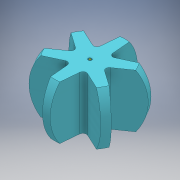
# Autodesk Inventor part: Dispensing Gear V2
Saved by Autodesk Inventor 2017 (Build 210142000, 142)
## iProperties
Created: 2018-12-12
Part Number: Dispensing Gear V2
Material: Generic
Document SubType Name: Modeling
Designer: Matt
Density: 1 g/cm^3
Appearance: Cadet Blue
Author: Matt
Autodesk Inventor part; units mm, degrees
ref_plane "YZ Plane" through (0, 0, 0) normal (1, 0, 0) x (0, 1, 0)
ref_plane "XZ Plane" through (0, 0, 0) normal (0, 1, 0) x (-1, 0, 0)
ref_plane "XY Plane" through (0, 0, 0) normal (0, 0, 1) x (1, 0, 0)
sketch "Sketch6" plane through (0, 0, 0) normal (0, 0, 1) x (1, 0, 0)
  circle A0 centre (0, 0) radius 2.75
  line L0 (0, 0) -> (0, 125)
  line L1 (0, 0) -> (108.2532, 62.5)
  line L2 (0, 0) -> (125, 0) construction
  line L3 (0, 0) -> (18.8687, 32.6815)
  line L4 (0, 0) -> (37.7374, 0) construction
  line L5 (108.2532, 62.5) -> (9.497, 16.4492)
  line L6 (108.2532, 62.5) -> (217.2186, 62.5) construction
  line L7 (9.497, 16.4492) -> (0, 125)
  line L8 (0, 125) -> (-9.497, 16.4492)
  line L9 (-9.497, 16.4492) -> (-108.2532, 62.5)
  line L10 (-108.2532, 62.5) -> (-18.9939, 0)
  line L11 (-18.9939, 0) -> (-108.2532, -62.5)
  line L12 (-108.2532, -62.5) -> (-9.497, -16.4492)
  line L13 (-9.497, -16.4492) -> (0, -125)
  line L14 (0, -125) -> (9.497, -16.4492)
  line L15 (9.497, -16.4492) -> (108.2532, -62.5)
  line L16 (108.2532, -62.5) -> (18.9939, 0)
  line L17 (18.9939, 0) -> (108.2532, 62.5)
  dimension "d21" = 5.5
  dimension "d22" = 125
  dimension "d23" = 30
  dimension "d24" = 60
  dimension "d25" = 155
  dimension "d28" = 360
  constraints: 36 end point, 3 equal length, 3 horizontal, 1 centre point, 1 coincident, 1 point on line, 1 vertical, 31 other
  measures "d21" diameter of A0
  measures "d22" distance of L0.start L0.end
  measures "d23" angle of L2 L1
  measures "d24" angle of L4 L3
  measures "d25" angle of L5 L6
extrude "Extrusion2" add sketch "Sketch6" along normal blind 76.2 contours L1 L3 A0 | A0 L3 L5 L1 | L0 L7 L3 A0 | A0 L3 L0
sketch "Sketch4" plane through (0, 0, 0) normal (0, 1, 0) x (-1, 0, 0)
  line L0 (-125.0691, 0) -> (-125.0691, 76.2)
  line L1 (0, -15.24) -> (0, 91.44) projected
  line L2 (-50.0691, 0) -> (-0.0691, 0)
  line L3 (-50, 76.2) -> (0, 76.2)
  line L4 (0, 76.2) -> (-125.0691, 76.2)
  line L5 (0, 0) -> (-108.2532, 0) projected
  line L6 (-125.0691, 0) -> (0, 0)
  arc A0 (-50, 76.2) -> (-50.0691, 0) centre (1.6634, 38.0531) ccw
  point P0 (-25, 76.2)
  point P1 (-0.0691, 76.2)
  point P2 (-62.5691, 76.2)
  dimension "d7" = 125
  dimension "d36" = 50
  dimension "d37" = 50
  constraints: 10 end point, 2 collinear, 2 point on circle, 1 centre point
  measures "d7" distance of L2.end L0.start
  measures "d36" distance of L2.start L2.end
  measures "d37" distance of L3.start L3.end
pattern_circular "Circular Pattern1" count 6 over 360 about axis through (0, 0, -10) along (0, 0, 1) of "Extrusion2"
revolve "Revolution2" cut sketch "Sketch4" angle 360 about axis through (0, 0, -10) along (0, 0, 1) contours L0 L4 A0 L5 L6
fillet "Fillet1" radius 5 1 edges at (-18.9939, 0, 38.1)
pattern_circular "Circular Pattern2" count 6 over 360 about axis through (0, 0, -10) along (0, 0, 1) of "Fillet1"
sketch "Sketch9" plane through (0, 0, 76.2) normal (0, 0, 1) x (1, 0, 0)
  circle A0 centre (0, 0) radius 2.5
  line L0 (0, 2.5) -> (0, 2.02)
  line L1 (0, 2.02) -> (-1.473, 2.02)
  line L2 (0, 2.02) -> (1.473, 2.02)
  dimension "d42" = 5
  dimension "d43" = 0.48
  constraints: 6 end point, 3 point on circle, 1 centre point, 1 coincident, 1 horizontal, 1 point on line, 1 vertical
  measures "d42" diameter of A0
  measures "d43" distance of L0.start L0.end
extrude "Extrusion3" cut sketch "Sketch9" against normal blind 14 contours A0 L1 L2
sketch "Sketch10" plane through (0, 0, 76.2) normal (0, 0, 1) x (1, 0, 0)
  point P0 (0, 0)
body "Solid1"
